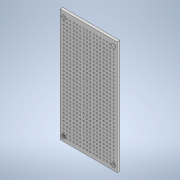
# Autodesk Inventor part: PCB2
Saved by Autodesk Inventor 2020 (Build 240168000, 168)
## iProperties
Created: 2020-06-09
Part Number: PCB2
Material: Generic
Document SubType Name: Modeling
Designer: Gebruiker
Density: 1 g/cm^3
Appearance: Default
Author: Gebruiker
Autodesk Inventor part; units mm, degrees
ref_plane "YZ Plane" through (0, 0, 0) normal (1, 0, 0) x (0, 1, 0)
ref_plane "XZ Plane" through (0, 0, 0) normal (0, 1, 0) x (-1, 0, 0)
ref_plane "XY Plane" through (0, 0, 0) normal (0, 0, 1) x (1, 0, 0)
sketch "Sketch1" plane through (0, 0, 0) normal (0, 0, 1) x (1, 0, 0)
  line L0 (-21.5, 42.5) -> (21.5, 42.5)
  line L1 (21.5, 42.5) -> (21.5, -42.5)
  line L2 (21.5, -42.5) -> (-21.5, -42.5)
  line L3 (-21.5, -42.5) -> (-21.5, 42.5)
  line L4 (-21.5, 42.5) -> (21.5, -42.5) construction
  line L5 (21.5, 42.5) -> (-21.5, -42.5) construction
  circle A0 centre (-18.75, 38.5) radius 0.5
  circle A1 centre (-18.75, 36) radius 0.5
  circle A2 centre (-18.75, 33.5) radius 0.5
  circle A3 centre (-18.75, 31) radius 0.5
  circle A4 centre (-18.75, 28.5) radius 0.5
  circle A5 centre (-18.75, 26) radius 0.5
  circle A6 centre (-18.75, 23.5) radius 0.5
  circle A7 centre (-18.75, 21) radius 0.5
  circle A8 centre (-18.75, 18.5) radius 0.5
  circle A9 centre (-18.75, 16) radius 0.5
  circle A10 centre (-18.75, 13.5) radius 0.5
  circle A11 centre (-18.75, 11) radius 0.5
  circle A12 centre (-18.75, 8.5) radius 0.5
  circle A13 centre (-18.75, 6) radius 0.5
  circle A14 centre (-18.75, 3.5) radius 0.5
  circle A15 centre (-18.75, 1) radius 0.5
  circle A16 centre (-18.75, -1.5) radius 0.5
  circle A17 centre (-18.75, -4) radius 0.5
  circle A18 centre (-18.75, -6.5) radius 0.5
  circle A19 centre (-18.75, -9) radius 0.5
  circle A20 centre (-18.75, -11.5) radius 0.5
  circle A21 centre (-18.75, -14) radius 0.5
  circle A22 centre (-18.75, -16.5) radius 0.5
  circle A23 centre (-18.75, -19) radius 0.5
  circle A24 centre (-18.75, -21.5) radius 0.5
  circle A25 centre (-18.75, -24) radius 0.5
  circle A26 centre (-18.75, -26.5) radius 0.5
  circle A27 centre (-18.75, -29) radius 0.5
  circle A28 centre (-18.75, -31.5) radius 0.5
  circle A29 centre (-18.75, -34) radius 0.5
  circle A30 centre (-18.75, -36.5) radius 0.5
  circle A31 centre (-18.75, -39) radius 0.5
  circle A32 centre (-16.25, 38.5) radius 0.5
  circle A33 centre (-16.25, 36) radius 0.5
  circle A34 centre (-16.25, 33.5) radius 0.5
  circle A35 centre (-16.25, 31) radius 0.5
  circle A36 centre (-16.25, 28.5) radius 0.5
  circle A37 centre (-16.25, 26) radius 0.5
  circle A38 centre (-16.25, 23.5) radius 0.5
  circle A39 centre (-16.25, 21) radius 0.5
  circle A40 centre (-16.25, 18.5) radius 0.5
  circle A41 centre (-16.25, 16) radius 0.5
  circle A42 centre (-16.25, 13.5) radius 0.5
  circle A43 centre (-16.25, 11) radius 0.5
  circle A44 centre (-16.25, 8.5) radius 0.5
  circle A45 centre (-16.25, 6) radius 0.5
  circle A46 centre (-16.25, 3.5) radius 0.5
  circle A47 centre (-16.25, 1) radius 0.5
  circle A48 centre (-16.25, -1.5) radius 0.5
  circle A49 centre (-16.25, -4) radius 0.5
  circle A50 centre (-16.25, -6.5) radius 0.5
  circle A51 centre (-16.25, -9) radius 0.5
  circle A52 centre (-16.25, -11.5) radius 0.5
  circle A53 centre (-16.25, -14) radius 0.5
  circle A54 centre (-16.25, -16.5) radius 0.5
  circle A55 centre (-16.25, -19) radius 0.5
  circle A56 centre (-16.25, -21.5) radius 0.5
  circle A57 centre (-16.25, -24) radius 0.5
  circle A58 centre (-16.25, -26.5) radius 0.5
  circle A59 centre (-16.25, -29) radius 0.5
  circle A60 centre (-16.25, -31.5) radius 0.5
  circle A61 centre (-16.25, -34) radius 0.5
  circle A62 centre (-16.25, -36.5) radius 0.5
  circle A63 centre (-16.25, -39) radius 0.5
  circle A64 centre (-13.75, 38.5) radius 0.5
  circle A65 centre (-13.75, 36) radius 0.5
  circle A66 centre (-13.75, 33.5) radius 0.5
  circle A67 centre (-13.75, 31) radius 0.5
  circle A68 centre (-13.75, 28.5) radius 0.5
  circle A69 centre (-13.75, 26) radius 0.5
  circle A70 centre (-13.75, 23.5) radius 0.5
  circle A71 centre (-13.75, 21) radius 0.5
  circle A72 centre (-13.75, 18.5) radius 0.5
  circle A73 centre (-13.75, 16) radius 0.5
  circle A74 centre (-13.75, 13.5) radius 0.5
  circle A75 centre (-13.75, 11) radius 0.5
  circle A76 centre (-13.75, 8.5) radius 0.5
  circle A77 centre (-13.75, 6) radius 0.5
  circle A78 centre (-13.75, 3.5) radius 0.5
  circle A79 centre (-13.75, 1) radius 0.5
  circle A80 centre (-13.75, -1.5) radius 0.5
  circle A81 centre (-13.75, -4) radius 0.5
  circle A82 centre (-13.75, -6.5) radius 0.5
  circle A83 centre (-13.75, -9) radius 0.5
  circle A84 centre (-13.75, -11.5) radius 0.5
  circle A85 centre (-13.75, -14) radius 0.5
  circle A86 centre (-13.75, -16.5) radius 0.5
  circle A87 centre (-13.75, -19) radius 0.5
  circle A88 centre (-13.75, -21.5) radius 0.5
  circle A89 centre (-13.75, -24) radius 0.5
  circle A90 centre (-13.75, -26.5) radius 0.5
  circle A91 centre (-13.75, -29) radius 0.5
  circle A92 centre (-13.75, -31.5) radius 0.5
  circle A93 centre (-13.75, -34) radius 0.5
  circle A94 centre (-13.75, -36.5) radius 0.5
  circle A95 centre (-13.75, -39) radius 0.5
  circle A96 centre (-11.25, 38.5) radius 0.5
  circle A97 centre (-11.25, 36) radius 0.5
  circle A98 centre (-11.25, 33.5) radius 0.5
  circle A99 centre (-11.25, 31) radius 0.5
  circle A100 centre (-11.25, 28.5) radius 0.5
  circle A101 centre (-11.25, 26) radius 0.5
  circle A102 centre (-11.25, 23.5) radius 0.5
  circle A103 centre (-11.25, 21) radius 0.5
  circle A104 centre (-11.25, 18.5) radius 0.5
  circle A105 centre (-11.25, 16) radius 0.5
  circle A106 centre (-11.25, 13.5) radius 0.5
  circle A107 centre (-11.25, 11) radius 0.5
  circle A108 centre (-11.25, 8.5) radius 0.5
  circle A109 centre (-11.25, 6) radius 0.5
  circle A110 centre (-11.25, 3.5) radius 0.5
  circle A111 centre (-11.25, 1) radius 0.5
  circle A112 centre (-11.25, -1.5) radius 0.5
  circle A113 centre (-11.25, -4) radius 0.5
  circle A114 centre (-11.25, -6.5) radius 0.5
  circle A115 centre (-11.25, -9) radius 0.5
  circle A116 centre (-11.25, -11.5) radius 0.5
  circle A117 centre (-11.25, -14) radius 0.5
  circle A118 centre (-11.25, -16.5) radius 0.5
  circle A119 centre (-11.25, -19) radius 0.5
  circle A120 centre (-11.25, -21.5) radius 0.5
  circle A121 centre (-11.25, -24) radius 0.5
  circle A122 centre (-11.25, -26.5) radius 0.5
  circle A123 centre (-11.25, -29) radius 0.5
  circle A124 centre (-11.25, -31.5) radius 0.5
  circle A125 centre (-11.25, -34) radius 0.5
  circle A126 centre (-11.25, -36.5) radius 0.5
  circle A127 centre (-11.25, -39) radius 0.5
  circle A128 centre (-8.75, 38.5) radius 0.5
  circle A129 centre (-8.75, 36) radius 0.5
  circle A130 centre (-8.75, 33.5) radius 0.5
  circle A131 centre (-8.75, 31) radius 0.5
  circle A132 centre (-8.75, 28.5) radius 0.5
  circle A133 centre (-8.75, 26) radius 0.5
  circle A134 centre (-8.75, 23.5) radius 0.5
  circle A135 centre (-8.75, 21) radius 0.5
  circle A136 centre (-8.75, 18.5) radius 0.5
  circle A137 centre (-8.75, 16) radius 0.5
  circle A138 centre (-8.75, 13.5) radius 0.5
  circle A139 centre (-8.75, 11) radius 0.5
  circle A140 centre (-8.75, 8.5) radius 0.5
  circle A141 centre (-8.75, 6) radius 0.5
  circle A142 centre (-8.75, 3.5) radius 0.5
  circle A143 centre (-8.75, 1) radius 0.5
  circle A144 centre (-8.75, -1.5) radius 0.5
  circle A145 centre (-8.75, -4) radius 0.5
  circle A146 centre (-8.75, -6.5) radius 0.5
  circle A147 centre (-8.75, -9) radius 0.5
  circle A148 centre (-8.75, -11.5) radius 0.5
  circle A149 centre (-8.75, -14) radius 0.5
  circle A150 centre (-8.75, -16.5) radius 0.5
  circle A151 centre (-8.75, -19) radius 0.5
  circle A152 centre (-8.75, -21.5) radius 0.5
  circle A153 centre (-8.75, -24) radius 0.5
  circle A154 centre (-8.75, -26.5) radius 0.5
  circle A155 centre (-8.75, -29) radius 0.5
  circle A156 centre (-8.75, -31.5) radius 0.5
  circle A157 centre (-8.75, -34) radius 0.5
  circle A158 centre (-8.75, -36.5) radius 0.5
  circle A159 centre (-8.75, -39) radius 0.5
  circle A160 centre (-6.25, 38.5) radius 0.5
  circle A161 centre (-6.25, 36) radius 0.5
  circle A162 centre (-6.25, 33.5) radius 0.5
  circle A163 centre (-6.25, 31) radius 0.5
  circle A164 centre (-6.25, 28.5) radius 0.5
  circle A165 centre (-6.25, 26) radius 0.5
  circle A166 centre (-6.25, 23.5) radius 0.5
  circle A167 centre (-6.25, 21) radius 0.5
  circle A168 centre (-6.25, 18.5) radius 0.5
  circle A169 centre (-6.25, 16) radius 0.5
  circle A170 centre (-6.25, 13.5) radius 0.5
  circle A171 centre (-6.25, 11) radius 0.5
  circle A172 centre (-6.25, 8.5) radius 0.5
  circle A173 centre (-6.25, 6) radius 0.5
  circle A174 centre (-6.25, 3.5) radius 0.5
  circle A175 centre (-6.25, 1) radius 0.5
  circle A176 centre (-6.25, -1.5) radius 0.5
  circle A177 centre (-6.25, -4) radius 0.5
  circle A178 centre (-6.25, -6.5) radius 0.5
  circle A179 centre (-6.25, -9) radius 0.5
  circle A180 centre (-6.25, -11.5) radius 0.5
  circle A181 centre (-6.25, -14) radius 0.5
  circle A182 centre (-6.25, -16.5) radius 0.5
  circle A183 centre (-6.25, -19) radius 0.5
  circle A184 centre (-6.25, -21.5) radius 0.5
  circle A185 centre (-6.25, -24) radius 0.5
  circle A186 centre (-6.25, -26.5) radius 0.5
  circle A187 centre (-6.25, -29) radius 0.5
  circle A188 centre (-6.25, -31.5) radius 0.5
  circle A189 centre (-6.25, -34) radius 0.5
  circle A190 centre (-6.25, -36.5) radius 0.5
  circle A191 centre (-6.25, -39) radius 0.5
  circle A192 centre (-3.75, 38.5) radius 0.5
  circle A193 centre (-3.75, 36) radius 0.5
  circle A194 centre (-3.75, 33.5) radius 0.5
  circle A195 centre (-3.75, 31) radius 0.5
  circle A196 centre (-3.75, 28.5) radius 0.5
  circle A197 centre (-3.75, 26) radius 0.5
  circle A198 centre (-3.75, 23.5) radius 0.5
  circle A199 centre (-3.75, 21) radius 0.5
  circle A200 centre (-3.75, 18.5) radius 0.5
  circle A201 centre (-3.75, 16) radius 0.5
  circle A202 centre (-3.75, 13.5) radius 0.5
  circle A203 centre (-3.75, 11) radius 0.5
  circle A204 centre (-3.75, 8.5) radius 0.5
  circle A205 centre (-3.75, 6) radius 0.5
  circle A206 centre (-3.75, 3.5) radius 0.5
  circle A207 centre (-3.75, 1) radius 0.5
  circle A208 centre (-3.75, -1.5) radius 0.5
  circle A209 centre (-3.75, -4) radius 0.5
  circle A210 centre (-3.75, -6.5) radius 0.5
  circle A211 centre (-3.75, -9) radius 0.5
  circle A212 centre (-3.75, -11.5) radius 0.5
  circle A213 centre (-3.75, -14) radius 0.5
  circle A214 centre (-3.75, -16.5) radius 0.5
  circle A215 centre (-3.75, -19) radius 0.5
  circle A216 centre (-3.75, -21.5) radius 0.5
  circle A217 centre (-3.75, -24) radius 0.5
  circle A218 centre (-3.75, -26.5) radius 0.5
  circle A219 centre (-3.75, -29) radius 0.5
  circle A220 centre (-3.75, -31.5) radius 0.5
  circle A221 centre (-3.75, -34) radius 0.5
  circle A222 centre (-3.75, -36.5) radius 0.5
  circle A223 centre (-3.75, -39) radius 0.5
  circle A224 centre (-1.25, 38.5) radius 0.5
  circle A225 centre (-1.25, 36) radius 0.5
  circle A226 centre (-1.25, 33.5) radius 0.5
  circle A227 centre (-1.25, 31) radius 0.5
  circle A228 centre (-1.25, 28.5) radius 0.5
  circle A229 centre (-1.25, 26) radius 0.5
  circle A230 centre (-1.25, 23.5) radius 0.5
  circle A231 centre (-1.25, 21) radius 0.5
  circle A232 centre (-1.25, 18.5) radius 0.5
  circle A233 centre (-1.25, 16) radius 0.5
  circle A234 centre (-1.25, 13.5) radius 0.5
  circle A235 centre (-1.25, 11) radius 0.5
  circle A236 centre (-1.25, 8.5) radius 0.5
  circle A237 centre (-1.25, 6) radius 0.5
  circle A238 centre (-1.25, 3.5) radius 0.5
  circle A239 centre (-1.25, 1) radius 0.5
  circle A240 centre (-1.25, -1.5) radius 0.5
  circle A241 centre (-1.25, -4) radius 0.5
  circle A242 centre (-1.25, -6.5) radius 0.5
  circle A243 centre (-1.25, -9) radius 0.5
  circle A244 centre (-1.25, -11.5) radius 0.5
  circle A245 centre (-1.25, -14) radius 0.5
  circle A246 centre (-1.25, -16.5) radius 0.5
  circle A247 centre (-1.25, -19) radius 0.5
  circle A248 centre (-1.25, -21.5) radius 0.5
  circle A249 centre (-1.25, -24) radius 0.5
  circle A250 centre (-1.25, -26.5) radius 0.5
  circle A251 centre (-1.25, -29) radius 0.5
  circle A252 centre (-1.25, -31.5) radius 0.5
  circle A253 centre (-1.25, -34) radius 0.5
  circle A254 centre (-1.25, -36.5) radius 0.5
  circle A255 centre (-1.25, -39) radius 0.5
  circle A256 centre (1.25, 38.5) radius 0.5
  circle A257 centre (1.25, 36) radius 0.5
  circle A258 centre (1.25, 33.5) radius 0.5
  circle A259 centre (1.25, 31) radius 0.5
  circle A260 centre (1.25, 28.5) radius 0.5
  circle A261 centre (1.25, 26) radius 0.5
  circle A262 centre (1.25, 23.5) radius 0.5
  circle A263 centre (1.25, 21) radius 0.5
  circle A264 centre (1.25, 18.5) radius 0.5
  circle A265 centre (1.25, 16) radius 0.5
  circle A266 centre (1.25, 13.5) radius 0.5
  circle A267 centre (1.25, 11) radius 0.5
  circle A268 centre (1.25, 8.5) radius 0.5
  circle A269 centre (1.25, 6) radius 0.5
  circle A270 centre (1.25, 3.5) radius 0.5
  circle A271 centre (1.25, 1) radius 0.5
  circle A272 centre (1.25, -1.5) radius 0.5
  circle A273 centre (1.25, -4) radius 0.5
  circle A274 centre (1.25, -6.5) radius 0.5
  circle A275 centre (1.25, -9) radius 0.5
  circle A276 centre (1.25, -11.5) radius 0.5
  circle A277 centre (1.25, -14) radius 0.5
  circle A278 centre (1.25, -16.5) radius 0.5
  circle A279 centre (1.25, -19) radius 0.5
  circle A280 centre (1.25, -21.5) radius 0.5
  circle A281 centre (1.25, -24) radius 0.5
  circle A282 centre (1.25, -26.5) radius 0.5
  circle A283 centre (1.25, -29) radius 0.5
  circle A284 centre (1.25, -31.5) radius 0.5
  circle A285 centre (1.25, -34) radius 0.5
  circle A286 centre (1.25, -36.5) radius 0.5
  circle A287 centre (1.25, -39) radius 0.5
  circle A288 centre (3.75, 38.5) radius 0.5
  circle A289 centre (3.75, 36) radius 0.5
  circle A290 centre (3.75, 33.5) radius 0.5
  circle A291 centre (3.75, 31) radius 0.5
  circle A292 centre (3.75, 28.5) radius 0.5
  circle A293 centre (3.75, 26) radius 0.5
  circle A294 centre (3.75, 23.5) radius 0.5
  circle A295 centre (3.75, 21) radius 0.5
  circle A296 centre (3.75, 18.5) radius 0.5
  circle A297 centre (3.75, 16) radius 0.5
  circle A298 centre (3.75, 13.5) radius 0.5
  circle A299 centre (3.75, 11) radius 0.5
  circle A300 centre (3.75, 8.5) radius 0.5
  circle A301 centre (3.75, 6) radius 0.5
  circle A302 centre (3.75, 3.5) radius 0.5
  circle A303 centre (3.75, 1) radius 0.5
  circle A304 centre (3.75, -1.5) radius 0.5
  circle A305 centre (3.75, -4) radius 0.5
  circle A306 centre (3.75, -6.5) radius 0.5
  circle A307 centre (3.75, -9) radius 0.5
  circle A308 centre (3.75, -11.5) radius 0.5
  circle A309 centre (3.75, -14) radius 0.5
  circle A310 centre (3.75, -16.5) radius 0.5
  circle A311 centre (3.75, -19) radius 0.5
  circle A312 centre (3.75, -21.5) radius 0.5
  circle A313 centre (3.75, -24) radius 0.5
  circle A314 centre (3.75, -26.5) radius 0.5
  circle A315 centre (3.75, -29) radius 0.5
  circle A316 centre (3.75, -31.5) radius 0.5
  circle A317 centre (3.75, -34) radius 0.5
  circle A318 centre (3.75, -36.5) radius 0.5
  circle A319 centre (3.75, -39) radius 0.5
  circle A320 centre (6.25, 38.5) radius 0.5
  circle A321 centre (6.25, 36) radius 0.5
  circle A322 centre (6.25, 33.5) radius 0.5
  circle A323 centre (6.25, 31) radius 0.5
  circle A324 centre (6.25, 28.5) radius 0.5
  circle A325 centre (6.25, 26) radius 0.5
  circle A326 centre (6.25, 23.5) radius 0.5
  circle A327 centre (6.25, 21) radius 0.5
  circle A328 centre (6.25, 18.5) radius 0.5
  circle A329 centre (6.25, 16) radius 0.5
  circle A330 centre (6.25, 13.5) radius 0.5
  circle A331 centre (6.25, 11) radius 0.5
  circle A332 centre (6.25, 8.5) radius 0.5
  circle A333 centre (6.25, 6) radius 0.5
  circle A334 centre (6.25, 3.5) radius 0.5
  circle A335 centre (6.25, 1) radius 0.5
  circle A336 centre (6.25, -1.5) radius 0.5
  circle A337 centre (6.25, -4) radius 0.5
  circle A338 centre (6.25, -6.5) radius 0.5
  circle A339 centre (6.25, -9) radius 0.5
  circle A340 centre (6.25, -11.5) radius 0.5
  circle A341 centre (6.25, -14) radius 0.5
  circle A342 centre (6.25, -16.5) radius 0.5
  circle A343 centre (6.25, -19) radius 0.5
  circle A344 centre (6.25, -21.5) radius 0.5
  circle A345 centre (6.25, -24) radius 0.5
  circle A346 centre (6.25, -26.5) radius 0.5
  circle A347 centre (6.25, -29) radius 0.5
  circle A348 centre (6.25, -31.5) radius 0.5
  circle A349 centre (6.25, -34) radius 0.5
  circle A350 centre (6.25, -36.5) radius 0.5
  circle A351 centre (6.25, -39) radius 0.5
  circle A352 centre (8.75, 38.5) radius 0.5
  circle A353 centre (8.75, 36) radius 0.5
  circle A354 centre (8.75, 33.5) radius 0.5
  circle A355 centre (8.75, 31) radius 0.5
  circle A356 centre (8.75, 28.5) radius 0.5
  circle A357 centre (8.75, 26) radius 0.5
  circle A358 centre (8.75, 23.5) radius 0.5
  circle A359 centre (8.75, 21) radius 0.5
  circle A360 centre (8.75, 18.5) radius 0.5
  circle A361 centre (8.75, 16) radius 0.5
  circle A362 centre (8.75, 13.5) radius 0.5
  circle A363 centre (8.75, 11) radius 0.5
  circle A364 centre (8.75, 8.5) radius 0.5
  circle A365 centre (8.75, 6) radius 0.5
  circle A366 centre (8.75, 3.5) radius 0.5
  circle A367 centre (8.75, 1) radius 0.5
  circle A368 centre (8.75, -1.5) radius 0.5
  circle A369 centre (8.75, -4) radius 0.5
  circle A370 centre (8.75, -6.5) radius 0.5
  circle A371 centre (8.75, -9) radius 0.5
  circle A372 centre (8.75, -11.5) radius 0.5
  circle A373 centre (8.75, -14) radius 0.5
  circle A374 centre (8.75, -16.5) radius 0.5
  circle A375 centre (8.75, -19) radius 0.5
  circle A376 centre (8.75, -21.5) radius 0.5
  circle A377 centre (8.75, -24) radius 0.5
  circle A378 centre (8.75, -26.5) radius 0.5
  circle A379 centre (8.75, -29) radius 0.5
  circle A380 centre (8.75, -31.5) radius 0.5
  circle A381 centre (8.75, -34) radius 0.5
  circle A382 centre (8.75, -36.5) radius 0.5
  circle A383 centre (8.75, -39) radius 0.5
  circle A384 centre (11.25, 38.5) radius 0.5
  circle A385 centre (11.25, 36) radius 0.5
  circle A386 centre (11.25, 33.5) radius 0.5
  circle A387 centre (11.25, 31) radius 0.5
  circle A388 centre (11.25, 28.5) radius 0.5
  circle A389 centre (11.25, 26) radius 0.5
  circle A390 centre (11.25, 23.5) radius 0.5
  circle A391 centre (11.25, 21) radius 0.5
  circle A392 centre (11.25, 18.5) radius 0.5
  circle A393 centre (11.25, 16) radius 0.5
  circle A394 centre (11.25, 13.5) radius 0.5
  circle A395 centre (11.25, 11) radius 0.5
  circle A396 centre (11.25, 8.5) radius 0.5
  circle A397 centre (11.25, 6) radius 0.5
  circle A398 centre (11.25, 3.5) radius 0.5
  circle A399 centre (11.25, 1) radius 0.5
  circle A400 centre (11.25, -1.5) radius 0.5
  circle A401 centre (11.25, -4) radius 0.5
  circle A402 centre (11.25, -6.5) radius 0.5
  circle A403 centre (11.25, -9) radius 0.5
  circle A404 centre (11.25, -11.5) radius 0.5
  circle A405 centre (11.25, -14) radius 0.5
  circle A406 centre (11.25, -16.5) radius 0.5
  circle A407 centre (11.25, -19) radius 0.5
  circle A408 centre (11.25, -21.5) radius 0.5
  circle A409 centre (11.25, -24) radius 0.5
  circle A410 centre (11.25, -26.5) radius 0.5
  circle A411 centre (11.25, -29) radius 0.5
  circle A412 centre (11.25, -31.5) radius 0.5
  circle A413 centre (11.25, -34) radius 0.5
  circle A414 centre (11.25, -36.5) radius 0.5
  circle A415 centre (11.25, -39) radius 0.5
  circle A416 centre (13.75, 38.5) radius 0.5
  circle A417 centre (13.75, 36) radius 0.5
  circle A418 centre (13.75, 33.5) radius 0.5
  circle A419 centre (13.75, 31) radius 0.5
  circle A420 centre (13.75, 28.5) radius 0.5
  circle A421 centre (13.75, 26) radius 0.5
  circle A422 centre (13.75, 23.5) radius 0.5
  circle A423 centre (13.75, 21) radius 0.5
  circle A424 centre (13.75, 18.5) radius 0.5
  circle A425 centre (13.75, 16) radius 0.5
  circle A426 centre (13.75, 13.5) radius 0.5
  circle A427 centre (13.75, 11) radius 0.5
  circle A428 centre (13.75, 8.5) radius 0.5
  circle A429 centre (13.75, 6) radius 0.5
  circle A430 centre (13.75, 3.5) radius 0.5
  circle A431 centre (13.75, 1) radius 0.5
  circle A432 centre (13.75, -1.5) radius 0.5
  circle A433 centre (13.75, -4) radius 0.5
  circle A434 centre (13.75, -6.5) radius 0.5
  circle A435 centre (13.75, -9) radius 0.5
  circle A436 centre (13.75, -11.5) radius 0.5
  circle A437 centre (13.75, -14) radius 0.5
  circle A438 centre (13.75, -16.5) radius 0.5
  circle A439 centre (13.75, -19) radius 0.5
  circle A440 centre (13.75, -21.5) radius 0.5
  circle A441 centre (13.75, -24) radius 0.5
  circle A442 centre (13.75, -26.5) radius 0.5
  circle A443 centre (13.75, -29) radius 0.5
  circle A444 centre (13.75, -31.5) radius 0.5
  circle A445 centre (13.75, -34) radius 0.5
  circle A446 centre (13.75, -36.5) radius 0.5
  circle A447 centre (13.75, -39) radius 0.5
  circle A448 centre (16.25, 38.5) radius 0.5
  circle A449 centre (16.25, 36) radius 0.5
  circle A450 centre (16.25, 33.5) radius 0.5
  circle A451 centre (16.25, 31) radius 0.5
  circle A452 centre (16.25, 28.5) radius 0.5
  circle A453 centre (16.25, 26) radius 0.5
  circle A454 centre (16.25, 23.5) radius 0.5
  circle A455 centre (16.25, 21) radius 0.5
  circle A456 centre (16.25, 18.5) radius 0.5
  circle A457 centre (16.25, 16) radius 0.5
  circle A458 centre (16.25, 13.5) radius 0.5
  circle A459 centre (16.25, 11) radius 0.5
  circle A460 centre (16.25, 8.5) radius 0.5
  circle A461 centre (16.25, 6) radius 0.5
  circle A462 centre (16.25, 3.5) radius 0.5
  circle A463 centre (16.25, 1) radius 0.5
  circle A464 centre (16.25, -1.5) radius 0.5
  circle A465 centre (16.25, -4) radius 0.5
  circle A466 centre (16.25, -6.5) radius 0.5
  circle A467 centre (16.25, -9) radius 0.5
  circle A468 centre (16.25, -11.5) radius 0.5
  circle A469 centre (16.25, -14) radius 0.5
  circle A470 centre (16.25, -16.5) radius 0.5
  circle A471 centre (16.25, -19) radius 0.5
  circle A472 centre (16.25, -21.5) radius 0.5
  circle A473 centre (16.25, -24) radius 0.5
  circle A474 centre (16.25, -26.5) radius 0.5
  circle A475 centre (16.25, -29) radius 0.5
  circle A476 centre (16.25, -31.5) radius 0.5
  circle A477 centre (16.25, -34) radius 0.5
  circle A478 centre (16.25, -36.5) radius 0.5
  circle A479 centre (16.25, -39) radius 0.5
  circle A480 centre (18.75, 38.5) radius 0.5
  circle A481 centre (18.75, 36) radius 0.5
  circle A482 centre (18.75, 33.5) radius 0.5
  circle A483 centre (18.75, 31) radius 0.5
  circle A484 centre (18.75, 28.5) radius 0.5
  circle A485 centre (18.75, 26) radius 0.5
  circle A486 centre (18.75, 23.5) radius 0.5
  circle A487 centre (18.75, 21) radius 0.5
  circle A488 centre (18.75, 18.5) radius 0.5
  circle A489 centre (18.75, 16) radius 0.5
  circle A490 centre (18.75, 13.5) radius 0.5
  circle A491 centre (18.75, 11) radius 0.5
  circle A492 centre (18.75, 8.5) radius 0.5
  circle A493 centre (18.75, 6) radius 0.5
  circle A494 centre (18.75, 3.5) radius 0.5
  circle A495 centre (18.75, 1) radius 0.5
  circle A496 centre (18.75, -1.5) radius 0.5
  circle A497 centre (18.75, -4) radius 0.5
  circle A498 centre (18.75, -6.5) radius 0.5
  circle A499 centre (18.75, -9) radius 0.5
  circle A500 centre (18.75, -11.5) radius 0.5
  circle A501 centre (18.75, -14) radius 0.5
  circle A502 centre (18.75, -16.5) radius 0.5
  circle A503 centre (18.75, -19) radius 0.5
  circle A504 centre (18.75, -21.5) radius 0.5
  circle A505 centre (18.75, -24) radius 0.5
  circle A506 centre (18.75, -26.5) radius 0.5
  circle A507 centre (18.75, -29) radius 0.5
  circle A508 centre (18.75, -31.5) radius 0.5
  circle A509 centre (18.75, -34) radius 0.5
  circle A510 centre (18.75, -36.5) radius 0.5
  circle A511 centre (18.75, -39) radius 0.5
  circle A512 centre (-18.75, 38.5) radius 1.5
  circle A513 centre (18.75, 38.5) radius 1.5
  circle A514 centre (-18.75, -39) radius 1.5
  circle A515 centre (18.75, -39) radius 1.5
  point P0 (0, 0)
  dimension "d0" = 43
  dimension "d1" = 85
  dimension "d2" = 1
  dimension "d3" = 3.5
  dimension "d4" = 2.75
  dimension "d23" = 2.5
  dimension "d26" = 2.5
  dimension "d29" = 3
  dimension "d30" = 3
  dimension "d31" = 3
  dimension "d32" = 3
  constraints: 516 centre point, 12 end point, 4 coincident, 2 horizontal, 2 midpoint, 2 parallel, 1 perpendicular, 1 vertical, 1022 other
  measures "d0" distance of L1.end L2.end
  measures "d1" distance of L0.end L1.end
  measures "d2" diameter of A0
  measures "d3" distance edge to line of A0 L0
  measures "d4" distance from line of L3 A0.centre
  measures "d23" distance of A0.centre A1.centre
  measures "d26" distance of A0.centre A32.centre
  measures "d29" diameter of A512
  measures "d30" diameter of A513
  measures "d31" diameter of A514
  measures "d32" diameter of A515
extrude "Extrusion1" add sketch "Sketch1" against normal blind 2 contours L0 L1 L2 L3
body "Solid1"
